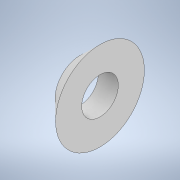
# Autodesk Inventor part: spacer
Saved by Autodesk Inventor 2022 (Build 260153000, 153)
## iProperties
Created: 2022-02-18
Part Number: spacer
Material: Genérico
Document SubType Name: Modeling
Designer: JK
Density: 1 g/cm^3
Appearance: Valor por defecto
Author: JK
Autodesk Inventor part; units mm, degrees
ref_plane "YZ Plane" through (0, 0, 0) normal (1, 0, 0) x (0, 1, 0)
ref_plane "XZ Plane" through (0, 0, 0) normal (0, 1, 0) x (-1, 0, 0)
ref_plane "XY Plane" through (0, 0, 0) normal (0, 0, 1) x (1, 0, 0)
sketch "Boceto2" plane through (0, 0, 0) normal (0, 1, 0) x (-1, 0, 0)
  line L0 (-0.7813, 0) -> (-0.7813, 2.25)
  line L1 (-0.7813, 2.25) -> (-2.5813, 4)
  line L2 (-2.5813, 4) -> (-2.5813, 0)
  line L3 (-2.5813, 0) -> (-0.7813, 0)
  line L4 (-0.7813, 1.65) -> (-2.5813, 1.65)
  point P0 (0, 0)
  dimension "d4" = 1.65
  dimension "d5" = 2.25
  dimension "d6" = 1.8
  dimension "d7" = 4
  constraints: 10 end point, 2 perpendicular, 2 point on line, 1 parallel, 1 vertical
  measures "d4" distance between parallel lines of L3 L4
  measures "d5" distance of L0.start L0.end
  measures "d6" distance between parallel lines of L2 L0
  measures "d7" distance of L2.end L1.end
revolve "Revolución1" add sketch "Boceto2" angle 360 about axis through (2.5813, 0, 0) along (-1, 0, 0) contours L4 L2 L1 L0
sketch "Boceto1" plane through (0, 0, 0) normal (0, 1, 0) x (-1, 0, 0)
  circle A0 centre (0, 0) radius 1.65
  circle A1 centre (0, 0) radius 2.25
  dimension "d0" = 3.3
  dimension "d1" = 4.5
  constraints: 2 centre point, 2 coincident
  measures "d0" diameter of A0
  measures "d1" diameter of A1
